Autodesk Inventor part; units mm, degrees
(part 2 of 3)
  line L883 (-85.6699, -58.7455) -> (-80.6699, -50.0853)
  line L884 (-66.3397, -69.9058) -> (-61.3397, -61.2455)
  line L885 (-61.3397, -61.2455) -> (-51.3397, -61.2455)
  line L886 (-51.3397, -61.2455) -> (-46.3397, -69.9058)
  line L887 (-51.3397, -61.2455) -> (-46.3397, -69.9058)
  line L888 (-51.3397, -78.566) -> (-61.3397, -78.566)
  line L889 (-51.3397, -78.566) -> (-61.3397, -78.566)
  line L890 (-61.3397, -78.566) -> (-66.3397, -69.9058)
  line L891 (-61.3397, -78.566) -> (-66.3397, -69.9058)
  line L892 (-46.3397, -69.9058) -> (-51.3397, -78.566)
  line L893 (-47.0096, -58.7455) -> (-42.0096, -50.0853)
  line L894 (-32.0096, -50.0853) -> (-27.0096, -58.7455)
  line L895 (-32.0096, -67.4058) -> (-42.0096, -67.4058)
  line L896 (-27.0096, -58.7455) -> (-32.0096, -67.4058)
  line L897 (-42.0096, -67.4058) -> (-47.0096, -58.7455)
  line L898 (-42.0096, -50.0853) -> (-32.0096, -50.0853)
  line L899 (-12.6795, -78.566) -> (-22.6795, -78.566)
  line L900 (-22.6795, -78.566) -> (-27.6795, -69.9058)
  line L901 (-27.6795, -69.9058) -> (-22.6795, -61.2455)
  line L902 (-7.6795, -69.9058) -> (-12.6795, -78.566)
  line L903 (-12.6795, -61.2455) -> (-7.6795, -69.9058)
  line L904 (-22.6795, -61.2455) -> (-12.6795, -61.2455)
  line L905 (25.981, -56.2455) -> (15.981, -56.2455)
  line L906 (15.981, -61.2455) -> (25.981, -61.2455)
  line L907 (6.6509, -67.4058) -> (-3.3491, -67.4058)
  line L908 (-3.3491, -67.4058) -> (-8.3491, -58.7455)
  line L909 (10.981, -69.9058) -> (15.981, -61.2455)
  line L910 (10.981, -69.9058) -> (15.981, -61.2455)
  line L911 (11.6509, -58.7455) -> (6.6509, -67.4058)
  line L912 (25.981, -61.2455) -> (30.981, -69.9058)
  line L913 (25.981, -61.2455) -> (30.981, -69.9058)
  line L914 (-8.3491, -58.7455) -> (-3.3491, -50.0853)
  line L915 (-3.3491, -50.0853) -> (6.6509, -50.0853)
  line L916 (6.6509, -50.0853) -> (11.6509, -58.7455)
  line L917 (54.6413, -78.566) -> (49.6413, -69.9058)
  line L918 (49.6413, -69.9058) -> (54.6413, -61.2455)
  line L919 (64.6413, -78.566) -> (54.6413, -78.566)
  line L920 (64.6413, -78.566) -> (54.6413, -78.566)
  line L921 (49.6413, -69.9058) -> (54.6413, -61.2455)
  line L922 (35.3111, -67.4058) -> (30.3111, -58.7455)
  line L923 (45.3111, -67.4058) -> (35.3111, -67.4058)
  line L924 (64.6413, -61.2455) -> (69.6413, -69.9058)
  line L925 (50.3111, -58.7455) -> (45.3111, -67.4058)
  line L926 (69.6413, -69.9058) -> (64.6413, -78.566)
  line L927 (73.9714, -72.4058) -> (83.9714, -72.4058)
  line L928 (83.9714, -67.4058) -> (73.9714, -67.4058)
  line L929 (73.9714, -67.4058) -> (68.9714, -58.7455)
  line L930 (45.3111, -50.0853) -> (50.3111, -58.7455)
  line L931 (68.9714, -58.7455) -> (73.9714, -50.0853)
  line L932 (93.3015, -78.566) -> (88.3015, -69.9058)
  line L933 (88.3015, -69.9058) -> (93.3015, -61.2455)
  line L934 (103.3015, -78.566) -> (93.3015, -78.566)
  line L935 (103.3015, -61.2455) -> (108.3015, -69.9058)
  line L936 (108.3015, -69.9058) -> (103.3015, -78.566)
  line L937 (54.6413, -61.2455) -> (64.6413, -61.2455)
  line L938 (73.9714, -50.0853) -> (83.9714, -50.0853)
  line L939 (35.3111, -50.0853) -> (45.3111, -50.0853)
  line L940 (30.3111, -58.7455) -> (35.3111, -50.0853)
  line L941 (15.981, -78.566) -> (10.981, -69.9058)
  line L942 (25.981, -78.566) -> (15.981, -78.566)
  line L943 (25.981, -78.566) -> (15.981, -78.566)
  line L944 (15.981, -78.566) -> (10.981, -69.9058)
  line L945 (69.6413, -69.9058) -> (64.6413, -78.566)
  line L946 (64.6413, -61.2455) -> (69.6413, -69.9058)
  line L947 (35.3111, -72.4058) -> (45.3111, -72.4058)
  line L948 (35.3111, -72.4058) -> (45.3111, -72.4058)
  line L949 (54.6413, -78.566) -> (49.6413, -69.9058)
  line L950 (30.981, -69.9058) -> (25.981, -78.566)
  line L951 (30.981, -69.9058) -> (25.981, -78.566)
  line L952 (103.3015, -56.2455) -> (93.3015, -56.2455)
  line L953 (107.6314, -58.7455) -> (112.6314, -50.0853)
  line L954 (112.6314, -50.0853) -> (122.6314, -50.0853)
  line L955 (112.6314, -67.4058) -> (107.6314, -58.7455)
  line L956 (122.6314, -50.0853) -> (127.6314, -58.7455)
  line L957 (122.6314, -67.4058) -> (112.6314, -67.4058)
  line L958 (127.6314, -58.7455) -> (122.6314, -67.4058)
  line L959 (93.3015, -61.2455) -> (103.3015, -61.2455)
  line L960 (88.9714, -58.7455) -> (83.9714, -67.4058)
  line L961 (83.9714, -50.0853) -> (88.9714, -58.7455)
  line L962 (-109.3301, -72.4063) -> (-104.3301, -81.0665)
  line L963 (-104.3301, -81.0665) -> (-109.3301, -89.7268)
  line L964 (-109.3301, -89.7268) -> (-119.3301, -89.7268)
  line L965 (-119.3301, -72.4063) -> (-109.3301, -72.4063)
  line L966 (-124.3301, -81.0665) -> (-119.3301, -72.4063)
  line L967 (-119.3301, -89.7268) -> (-124.3301, -81.0665)
  line L968 (-105, -92.2268) -> (-100, -83.5665)
  line L969 (-100, -83.5665) -> (-90, -83.5665)
  line L970 (-90, -83.5665) -> (-85, -92.2268)
  line L971 (-85, -92.2268) -> (-90, -100.887)
  line L972 (-90, -100.887) -> (-100, -100.887)
  line L973 (-100, -100.887) -> (-105, -92.2268)
  line L974 (-80.6699, -89.7268) -> (-85.6699, -81.0665)
  line L975 (-65.6699, -81.0665) -> (-70.6699, -89.7268)
  line L976 (-70.6699, -72.4063) -> (-65.6699, -81.0665)
  line L977 (-80.6699, -72.4063) -> (-70.6699, -72.4063)
  line L978 (-70.6699, -89.7268) -> (-80.6699, -89.7268)
  line L979 (-85.6699, -81.0665) -> (-80.6699, -72.4063)
  line L980 (-66.3397, -92.2268) -> (-61.3397, -83.5665)
  line L981 (-61.3397, -83.5665) -> (-51.3397, -83.5665)
  line L982 (-51.3397, -83.5665) -> (-46.3397, -92.2268)
  line L983 (-51.3397, -83.5665) -> (-46.3397, -92.2268)
  line L984 (-51.3397, -100.887) -> (-61.3397, -100.887)
  line L985 (-51.3397, -100.887) -> (-61.3397, -100.887)
  line L986 (-61.3397, -100.887) -> (-66.3397, -92.2268)
  line L987 (-61.3397, -100.887) -> (-66.3397, -92.2268)
  line L988 (-46.3397, -92.2268) -> (-51.3397, -100.887)
  line L989 (-47.0096, -81.0665) -> (-42.0096, -72.4063)
  line L990 (-32.0096, -72.4063) -> (-27.0096, -81.0665)
  line L991 (-32.0096, -89.7268) -> (-42.0096, -89.7268)
  line L992 (-27.0096, -81.0665) -> (-32.0096, -89.7268)
  line L993 (-42.0096, -89.7268) -> (-47.0096, -81.0665)
  line L994 (-42.0096, -72.4063) -> (-32.0096, -72.4063)
  line L995 (-12.6795, -100.887) -> (-22.6795, -100.887)
  line L996 (-22.6795, -100.887) -> (-27.6795, -92.2268)
  line L997 (-27.6795, -92.2268) -> (-22.6795, -83.5665)
  line L998 (-7.6795, -92.2268) -> (-12.6795, -100.887)
  line L999 (-12.6795, -83.5665) -> (-7.6795, -92.2268)
  line L1000 (-22.6795, -83.5665) -> (-12.6795, -83.5665)
  line L1001 (25.981, -78.5665) -> (15.981, -78.5665)
  line L1002 (15.981, -83.5665) -> (25.981, -83.5665)
  line L1003 (6.6509, -89.7268) -> (-3.3491, -89.7268)
  line L1004 (-3.3491, -89.7268) -> (-8.3491, -81.0665)
  line L1005 (10.981, -92.2268) -> (15.981, -83.5665)
  line L1006 (10.981, -92.2268) -> (15.981, -83.5665)
  line L1007 (11.6509, -81.0665) -> (6.6509, -89.7268)
  line L1008 (25.981, -83.5665) -> (30.981, -92.2268)
  line L1009 (25.981, -83.5665) -> (30.981, -92.2268)
  line L1010 (-8.3491, -81.0665) -> (-3.3491, -72.4063)
  line L1011 (-3.3491, -72.4063) -> (6.6509, -72.4063)
  line L1012 (6.6509, -72.4063) -> (11.6509, -81.0665)
  line L1013 (54.6413, -100.887) -> (49.6413, -92.2268)
  line L1014 (49.6413, -92.2268) -> (54.6413, -83.5665)
  line L1015 (64.6413, -100.887) -> (54.6413, -100.887)
  line L1016 (64.6413, -100.887) -> (54.6413, -100.887)
  line L1017 (49.6413, -92.2268) -> (54.6413, -83.5665)
  line L1018 (35.3111, -89.7268) -> (30.3111, -81.0665)
  line L1019 (45.3111, -89.7268) -> (35.3111, -89.7268)
  line L1020 (64.6413, -83.5665) -> (69.6413, -92.2268)
  line L1021 (50.3111, -81.0665) -> (45.3111, -89.7268)
  line L1022 (69.6413, -92.2268) -> (64.6413, -100.887)
  line L1023 (73.9714, -94.7268) -> (83.9714, -94.7268)
  line L1024 (83.9714, -89.7268) -> (73.9714, -89.7268)
  line L1025 (73.9714, -89.7268) -> (68.9714, -81.0665)
  line L1026 (45.3111, -72.4063) -> (50.3111, -81.0665)
  line L1027 (68.9714, -81.0665) -> (73.9714, -72.4063)
  line L1028 (93.3015, -100.887) -> (88.3015, -92.2268)
  line L1029 (88.3015, -92.2268) -> (93.3015, -83.5665)
  line L1030 (103.3015, -100.887) -> (93.3015, -100.887)
  line L1031 (103.3015, -83.5665) -> (108.3015, -92.2268)
  line L1032 (108.3015, -92.2268) -> (103.3015, -100.887)
  line L1033 (54.6413, -83.5665) -> (64.6413, -83.5665)
  line L1034 (73.9714, -72.4063) -> (83.9714, -72.4063)
  line L1035 (35.3111, -72.4063) -> (45.3111, -72.4063)
  line L1036 (30.3111, -81.0665) -> (35.3111, -72.4063)
  line L1037 (15.981, -100.887) -> (10.981, -92.2268)
  line L1038 (25.981, -100.887) -> (15.981, -100.887)
  line L1039 (25.981, -100.887) -> (15.981, -100.887)
  line L1040 (15.981, -100.887) -> (10.981, -92.2268)
  line L1041 (69.6413, -92.2268) -> (64.6413, -100.887)
  line L1042 (64.6413, -83.5665) -> (69.6413, -92.2268)
  line L1043 (35.3111, -94.7268) -> (45.3111, -94.7268)
  line L1044 (35.3111, -94.7268) -> (45.3111, -94.7268)
  line L1045 (54.6413, -100.887) -> (49.6413, -92.2268)
  line L1046 (30.981, -92.2268) -> (25.981, -100.887)
  line L1047 (30.981, -92.2268) -> (25.981, -100.887)
  line L1048 (103.3015, -78.5665) -> (93.3015, -78.5665)
  line L1049 (107.6314, -81.0665) -> (112.6314, -72.4063)
  line L1050 (112.6314, -72.4063) -> (122.6314, -72.4063)
  line L1051 (112.6314, -89.7268) -> (107.6314, -81.0665)
  line L1052 (122.6314, -72.4063) -> (127.6314, -81.0665)
  line L1053 (122.6314, -89.7268) -> (112.6314, -89.7268)
  line L1054 (127.6314, -81.0665) -> (122.6314, -89.7268)
  line L1055 (93.3015, -83.5665) -> (103.3015, -83.5665)
  line L1056 (88.9714, -81.0665) -> (83.9714, -89.7268)
  line L1057 (83.9714, -72.4063) -> (88.9714, -81.0665)
  line L1058 (-109.3301, -94.7273) -> (-104.3301, -103.3875)
  line L1059 (-104.3301, -103.3875) -> (-109.3301, -112.0478)
  line L1060 (-109.3301, -112.0478) -> (-119.3301, -112.0478)
  line L1061 (-119.3301, -94.7273) -> (-109.3301, -94.7273)
  line L1062 (-124.3301, -103.3875) -> (-119.3301, -94.7273)
  line L1063 (-119.3301, -112.0478) -> (-124.3301, -103.3875)
  line L1064 (-105, -114.5478) -> (-100, -105.8875)
  line L1065 (-100, -105.8875) -> (-90, -105.8875)
  line L1066 (-90, -105.8875) -> (-85, -114.5478)
  line L1067 (-85, -114.5478) -> (-90, -123.208)
  line L1068 (-90, -123.208) -> (-100, -123.208)
  line L1069 (-100, -123.208) -> (-105, -114.5478)
  line L1070 (-80.6699, -112.0478) -> (-85.6699, -103.3875)
  line L1071 (-65.6699, -103.3875) -> (-70.6699, -112.0478)
  line L1072 (-70.6699, -94.7273) -> (-65.6699, -103.3875)
  line L1073 (-80.6699, -94.7273) -> (-70.6699, -94.7273)
  line L1074 (-70.6699, -112.0478) -> (-80.6699, -112.0478)
  line L1075 (-85.6699, -103.3875) -> (-80.6699, -94.7273)
  line L1076 (-66.3397, -114.5478) -> (-61.3397, -105.8875)
  line L1077 (-61.3397, -105.8875) -> (-51.3397, -105.8875)
  line L1078 (-51.3397, -105.8875) -> (-46.3397, -114.5478)
  line L1079 (-51.3397, -105.8875) -> (-46.3397, -114.5478)
  line L1080 (-51.3397, -123.208) -> (-61.3397, -123.208)
  line L1081 (-51.3397, -123.208) -> (-61.3397, -123.208)
  line L1082 (-61.3397, -123.208) -> (-66.3397, -114.5478)
  line L1083 (-61.3397, -123.208) -> (-66.3397, -114.5478)
  line L1084 (-46.3397, -114.5478) -> (-51.3397, -123.208)
  line L1085 (-47.0096, -103.3875) -> (-42.0096, -94.7273)
  line L1086 (-32.0096, -94.7273) -> (-27.0096, -103.3875)
  line L1087 (-32.0096, -112.0478) -> (-42.0096, -112.0478)
  line L1088 (-27.0096, -103.3875) -> (-32.0096, -112.0478)
  line L1089 (-42.0096, -112.0478) -> (-47.0096, -103.3875)
  line L1090 (-42.0096, -94.7273) -> (-32.0096, -94.7273)
  line L1091 (-12.6795, -123.208) -> (-22.6795, -123.208)
  line L1092 (-22.6795, -123.208) -> (-27.6795, -114.5478)
  line L1093 (-27.6795, -114.5478) -> (-22.6795, -105.8875)
  line L1094 (-7.6795, -114.5478) -> (-12.6795, -123.208)
  line L1095 (-12.6795, -105.8875) -> (-7.6795, -114.5478)
  line L1096 (-22.6795, -105.8875) -> (-12.6795, -105.8875)
  line L1097 (25.981, -100.8875) -> (15.981, -100.8875)
  line L1098 (15.981, -105.8875) -> (25.981, -105.8875)
  line L1099 (6.6509, -112.0478) -> (-3.3491, -112.0478)
  line L1100 (-3.3491, -112.0478) -> (-8.3491, -103.3875)
  line L1101 (10.981, -114.5478) -> (15.981, -105.8875)
  line L1102 (10.981, -114.5478) -> (15.981, -105.8875)
  line L1103 (11.6509, -103.3875) -> (6.6509, -112.0478)
  line L1104 (25.981, -105.8875) -> (30.981, -114.5478)
  line L1105 (25.981, -105.8875) -> (30.981, -114.5478)
  line L1106 (-8.3491, -103.3875) -> (-3.3491, -94.7273)
  line L1107 (-3.3491, -94.7273) -> (6.6509, -94.7273)
  line L1108 (6.6509, -94.7273) -> (11.6509, -103.3875)
  line L1109 (54.6413, -123.208) -> (49.6413, -114.5478)
  line L1110 (49.6413, -114.5478) -> (54.6413, -105.8875)
  line L1111 (64.6413, -123.208) -> (54.6413, -123.208)
  line L1112 (64.6413, -123.208) -> (54.6413, -123.208)
  line L1113 (49.6413, -114.5478) -> (54.6413, -105.8875)
  line L1114 (35.3111, -112.0478) -> (30.3111, -103.3875)
  line L1115 (45.3111, -112.0478) -> (35.3111, -112.0478)
  line L1116 (64.6413, -105.8875) -> (69.6413, -114.5478)
  line L1117 (50.3111, -103.3875) -> (45.3111, -112.0478)
  line L1118 (69.6413, -114.5478) -> (64.6413, -123.208)
  line L1119 (73.9714, -117.0478) -> (83.9714, -117.0478)
  line L1120 (83.9714, -112.0478) -> (73.9714, -112.0478)
  line L1121 (73.9714, -112.0478) -> (68.9714, -103.3875)
  line L1122 (45.3111, -94.7273) -> (50.3111, -103.3875)
  line L1123 (68.9714, -103.3875) -> (73.9714, -94.7273)
  line L1124 (93.3015, -123.208) -> (88.3015, -114.5478)
  line L1125 (88.3015, -114.5478) -> (93.3015, -105.8875)
  line L1126 (103.3015, -123.208) -> (93.3015, -123.208)
  line L1127 (103.3015, -105.8875) -> (108.3015, -114.5478)
  line L1128 (108.3015, -114.5478) -> (103.3015, -123.208)
  line L1129 (54.6413, -105.8875) -> (64.6413, -105.8875)
  line L1130 (73.9714, -94.7273) -> (83.9714, -94.7273)
  line L1131 (35.3111, -94.7273) -> (45.3111, -94.7273)
  line L1132 (30.3111, -103.3875) -> (35.3111, -94.7273)
  line L1133 (15.981, -123.208) -> (10.981, -114.5478)
  line L1134 (25.981, -123.208) -> (15.981, -123.208)
  line L1135 (25.981, -123.208) -> (15.981, -123.208)
  line L1136 (15.981, -123.208) -> (10.981, -114.5478)
  line L1137 (69.6413, -114.5478) -> (64.6413, -123.208)
  line L1138 (64.6413, -105.8875) -> (69.6413, -114.5478)
  line L1139 (35.3111, -117.0478) -> (45.3111, -117.0478)
  line L1140 (35.3111, -117.0478) -> (45.3111, -117.0478)
  line L1141 (54.6413, -123.208) -> (49.6413, -114.5478)
  line L1142 (30.981, -114.5478) -> (25.981, -123.208)
  line L1143 (30.981, -114.5478) -> (25.981, -123.208)
  line L1144 (103.3015, -100.8875) -> (93.3015, -100.8875)
  line L1145 (107.6314, -103.3875) -> (112.6314, -94.7273)
  line L1146 (112.6314, -94.7273) -> (122.6314, -94.7273)
  line L1147 (112.6314, -112.0478) -> (107.6314, -103.3875)
  line L1148 (122.6314, -94.7273) -> (127.6314, -103.3875)
  line L1149 (122.6314, -112.0478) -> (112.6314, -112.0478)
  line L1150 (127.6314, -103.3875) -> (122.6314, -112.0478)
  line L1151 (93.3015, -105.8875) -> (103.3015, -105.8875)
  line L1152 (88.9714, -103.3875) -> (83.9714, -112.0478)
  line L1153 (83.9714, -94.7273) -> (88.9714, -103.3875)
  point P0 (0, 0)
  point P1 (-100, 79)
  point P2 (-100, 71.25)
  point P3 (-100, 86.75)
  point P4 (-60, 79)
  point P5 (-60, 71.25)
  point P6 (-60, 86.75)
  point P7 (-20, 79)
  point P8 (-20, 71.25)
  point P9 (-20, 86.75)
  point P10 (20, 79)
  point P11 (20, 71.25)
  point P12 (20, 86.75)
  point P13 (60, 79)
  point P14 (60, 71.25)
  point P15 (60, 86.75)
  point P16 (100, 79)
  point P17 (100, 71.25)
  point P18 (100, 86.75)
  point P19 (100, 79)
  point P20 (-80, 39.5)
  point P21 (-80, 47.25)
  point P22 (-80, 31.75)
  point P23 (-40, 47.25)
  point P24 (-40, 39.5)
  point P25 (-40, 31.75)
  point P26 (0, 47.25)
  point P27 (0, 39.5)
  point P28 (0, 31.75)
  point P29 (40, 47.25)
  point P30 (40, 39.5)
  point P31 (40, 31.75)
  point P32 (80, 47.25)
  point P33 (80, 39.5)
  point P34 (80, 31.75)
  point P35 (-100, 0)
  point P36 (-100, -7.75)
  point P37 (-100, 7.75)
  point P38 (-60, 0)
  point P39 (-60, -7.75)
  point P40 (-60, 7.75)
  point P41 (-20, 0)
  point P42 (-20, -7.75)
  point P43 (-20, 7.75)
  point P44 (20, 0)
  point P45 (20, -7.75)
  point P46 (20, 7.75)
  point P47 (60, 0)
  point P48 (60, -7.75)
  point P49 (60, 7.75)
  point P50 (100, 0)
  point P51 (100, 0)
  point P52 (100, -7.75)
  point P53 (100, 7.75)
  point P54 (-100, -79)
  point P55 (-100, -86.75)
  point P56 (-100, -71.25)
  point P57 (-60, -79)
  point P58 (-60, -86.75)
  point P59 (-60, -71.25)
  point P60 (-20, -79)
  point P61 (-20, -86.75)
  point P62 (-20, -71.25)
  point P63 (20, -79)
  point P64 (20, -86.75)
  point P65 (20, -71.25)
  point P66 (60, -79)
  point P67 (60, -86.75)
  point P68 (60, -71.25)
  point P69 (100, -79)
  point P70 (100, -79)
  point P71 (100, -86.75)
  point P72 (100, -71.25)
  point P73 (-80, -39.5)
  point P74 (-80, -47.25)
  point P75 (-80, -31.75)
  point P76 (0, -31.75)
  point P77 (0, -39.5)
  point P78 (0, -47.25)
  point P79 (40, -31.75)
  point P80 (40, -39.5)
  point P81 (40, -47.25)
  point P82 (80, -31.75)
  point P83 (80, -39.5)
  point P84 (80, -47.25)
  point P85 (-40, -31.75)
  point P86 (-40, -39.5)
  point P87 (-40, -47.25)
  point P88 (100, -86.75)
  point P89 (-60, -86.75)
  point P90 (60, 79)
  point P91 (-95, 86.3397)
  point P92 (-95, 95)
  point P93 (-75.6699, 75.1795)
  point P94 (-75.6699, 83.8397)
  point P95 (-75.6699, 97.5)
  point P96 (-174.6517, 120.5465)
  point P97 (-114.3301, 97.5)
  point P98 (-95, 108.6603)
  point P99 (-102.5, 68.3494)
  point P100 (-83.1699, 48.5289)
  point P101 (-56.3397, 55.359)
  point P102 (-48.8397, 82.0096)
  point P103 (-68.1699, 101.8301)
  point P104 (-114.3301, 75.1795)
  point P105 (-37.0096, 75.1795)
  point P106 (-44.5096, 70.8494)
  point P107 (-29.5096, 48.5289)
  point P108 (-10.1795, 68.3494)
  point P109 (-17.6795, 95)
  point P110 (-44.5096, 101.8301)
  point P111 (20.981, 95)
  point P112 (40.3111, 75.1795)
  point P113 (32.8111, 48.5289)
  point P114 (40.3111, 83.8397)
  point P115 (40.3111, 97.5)
  point P116 (47.8111, 101.8301)
  point P117 (13.481, 68.3494)
  point P118 (20.981, 108.6603)
  point P119 (1.6509, 75.1795)
  point P120 (1.6509, 97.5)
  point P121 (59.6413, 55.359)
  point P122 (67.1413, 82.0096)
  point P123 (71.4714, 101.8301)
  point P124 (78.9714, 75.1795)
  point P125 (71.4714, 70.8494)
  point P126 (86.4714, 48.5289)
  point P127 (98.3015, 95)
  point P128 (105.8015, 68.3494)
  point P129 (117.6314, 75.1795)
  point P130 (98.3014, 33.0387)
  point P131 (98.3014, 41.6989)
  point P132 (144.4614, 37.3688)
  point P133 (136.9614, 41.6989)
  point P134 (163.7914, 79.5096)
  point P135 (156.2914, 75.1795)
  point P136 (136.9614, 117.3203)
  point P137 (136.9614, 108.66)
  point P138 (90.8014, 112.9902)
  point P139 (98.3014, 108.66)
  point P140 (70, 33.038)
  point P141 (86.4714, -18.4331)
  point P142 (93.3014, -16.6028)
  point P143 (103.3014, -16.6028)
  point P144 (78.9714, 8.2175)
  point P145 (71.4714, 3.8874)
  point P146 (59.6413, -11.603)
  point P147 (105.8015, 1.3874)
  point P148 (100, 12.038)
  point P149 (117.6314, 8.2175)
  point P150 (67.1413, 15.0476)
  point P151 (32.8111, -18.4331)
  point P152 (40.3111, 8.2175)
  point P153 (13.481, 1.3874)
  point P154 (98.3014, 41.698)
  point P155 (98.3015, 28.038)
  point P156 (40.3111, 16.8777)
  point P157 (71.4714, 34.8681)
  point P158 (90.8014, 46.0282)
  point P159 (40.3111, 30.538)
  point P160 (47.8111, 34.8681)
  point P161 (20.981, 28.038)
  point P162 (20.981, 41.6983)
  point P163 (-48.8397, 15.0476)
  point P164 (1.6509, 8.2175)
  point P165 (-83.1699, -18.4331)
  point P166 (-29.5096, -18.4331)
  point P167 (1.6509, 30.538)
  point P168 (-10.1795, 1.3874)
  point P169 (-44.5096, 3.8874)
  point P170 (-37.0096, 8.2175)
  point P171 (-17.6795, 28.038)
  point P172 (-44.5096, 34.8681)
  point P173 (-68.1699, 34.8681)
  point P174 (-75.6699, 8.2175)
  point P175 (-56.3397, -11.603)
  point P176 (-75.6699, 30.538)
  point P177 (-75.6699, 16.8777)
  point P178 (-95, 28.038)
  point P179 (-95, 19.3777)
  point P180 (-95, 41.6983)
  point P181 (-102.5, 1.3874)
  point P182 (-114.3301, 8.2175)
  point P183 (-114.3301, 30.538)
  point P184 (0, -66.962)
  point P185 (-56.3399, 41.6985)
  point P186 (-17.6795, 41.6985)
  point P187 (1.6509, 52.859)
  point P188 (59.6413, 41.6983)
  point P189 (-68.1699, 48.5289)
  point P190 (-114.3301, 52.859)
  point P191 (-114.3301, -14.1035)
  point P192 (-102.5, -20.9336)
  point P193 (-75.6699, -14.1035)
  point P194 (-75.6699, -5.4433)
  point P195 (-56.3397, -33.924)
  point P196 (-44.5096, -18.4336)
  point P197 (-37.0096, -14.1035)
  point P198 (-46.3397, -2.9433)
  point P199 (-46.3397, -2.9433)
  dimension "d0" = 220
  dimension "d1" = 200
  dimension "d2" = 5.5
  dimension "d3" = 15.5
  dimension "d7" = 10
  dimension "d8" = 21
  dimension "d13" = 40
  dimension "d20" = 5.5
  dimension "d21" = 15.5
  dimension "d22" = 30
  dimension "d24" = 55
  dimension "d30" = 40
  dimension "d37" = 79
  dimension "d44" = 79
  dimension "d51" = 13.25
  dimension "d52" = 13.25
  dimension "d76" = 180
  dimension "d77" = 10
  dimension "d159" = 20
  dimension "d160" = 5
  dimension "d161" = 5
  dimension "d162" = 20
  dimension "d164" = 5
  dimension "d166" = 20
  dimension "d167" = 5
  dimension "d168" = 5
  dimension "d170" = 20
  dimension "d171" = 5
  dimension "d172" = 20
  dimension "d173" = 5
  dimension "d174" = 5
  dimension "d175" = 5
  dimension "d178" = 360
  dimension "d182" = 60
  dimension "d184" = 20
  dimension "d185" = 5
  dimension "d186" = 5
  dimension "d189" = 240
  dimension "d193" = 115.981
  dimension "d198" = 20
  dimension "d199" = 38.6602
  dimension "d200" = 38.66
  dimension "d203" = 360
  dimension "d207" = 66.962
  dimension "d212" = 5.0005
  dimension "d213" = 20
  dimension "d214" = 5
  dimension "d215" = 5
  dimension "d216" = 20
  dimension "d217" = 20
  dimension "d218" = 20
  dimension "d219" = 20
  dimension "d222" = 22.321
  constraints: 2358 end point, 1202 vertical alignment, 738 parallel, 118 point on circle, 56 centre point, 51 collinear, 34 equal radius, 18 horizontal, 10 midpoint, 8 tangent, 6 horizontal alignment, 4 vertical, 1 perpendicular, 1 point on line, 899 other
  measures "d0" distance of L1.end L2.end
  measures "d1" distance of L1.start L1.end
  measures "d2" distance between parallel lines of L8 L7
  measures "d3" distance of point (-100, 71.25) point (-100, 86.75)
  measures "d8" distance from line of L2 point (-100, 79)
  measures "d13" distance of L7.start L9.start
  measures "d20" distance between parallel lines of L26 L25
  measures "d21" distance of point (-80, 47.25) point (-80, 31.75)
  measures "d24" vertical distance of point (-80, 31.75) point (-100, 86.75)
  measures "d30" distance of point (-80, 47.25) point (-40, 47.25)
  measures "d37" distance of point (-100, 79) point (-100, 0)
  measures "d44" distance of L24.start L75.start
  measures "d52" distance from line of L2 point (-100, 86.75)
  measures "d77" distance from line of L90 point (60, 79)
  measures "d159" distance of L91.start L93.end
  measures "d161" distance from line of L2 point (-95, 95)
  measures "d162" distance of L100.end L97.end
  measures "d164" distance between parallel lines of L91 L98
  measures "d166" distance of L105.start L107.end
  measures "d167" distance between parallel lines of L107 L96
  measures "d168" distance between parallel lines of L99 L106
  measures "d170" distance of L121.end L117.end
  measures "d171" distance between parallel lines of L94 L119
  measures "d172" distance of L125.start L123.end
  measures "d173" distance between parallel lines of L95 L124
  measures "d174" distance between parallel lines of L108 L125
  measures "d175" distance between parallel lines of L123 L121
  measures "d184" distance of L197.start L195.end
  measures "d185" distance from line of point (-44.51, 70.849) L154
  measures "d186" distance between parallel lines of L200 L187
  measures "d193" distance of L107.end L245.end
  measures "d198" distance of L353.start L351.end
  measures "d199" distance of point (40.311, 75.179) point (78.971, 75.179)
  measures "d200" distance of point (117.631, 75.179) point (78.971, 75.179)
  measures "d207" distance of L1.end L626.end
  measures "d212" distance between parallel lines of L130 L603
  measures "d213" distance of L646.start L644.end
  measures "d214" distance from line of point (-68.17, 48.529) L649
  measures "d215" distance between parallel lines of L565 L644
  measures "d216" distance of L652.start L650.end
  measures "d217" distance of L658.start L656.end
  measures "d218" distance of L662.end L664.start
  measures "d219" distance of L670.start L668.end
  measures "d222" distance of L609.start L674.start
extrude "돌출1" add sketch "스케치1" along normal blind 5 contours L3 L1061 L1058 L0 | L1058 L1061 L3 L964 L963 L962 L965 L868 L867 L866 L869 L772 L771 L770 L773 L676 L675 L674 L677 L608 L607 L609 L610 L615 L614 L613 L387 L583 L584 L588 L564 L565 L562 L560 L557 L558 L559 L537 L539 L538 L536 L535 L486 L465 L464 L484 L488 L90 L472 L473 L435 L396 L391 L390 L835 L833 L931 L929 L1027 L1025 L0 L1022 L1020 L1033 L71 L919 L926 L924 L937 L918 L917 L69 L1014 L1013 L1122 L1043 L1132 L1046 L1008 L1002 L68 L942 L950 L912 L906 L909 L941 L66 L1005 L1037 L1108 L1107 L1106 L998 L999 L1000 L65 L899 L902 L903 L904 L901 L900 L63 L997 L996 L1086 L1090 L1085 L988 L982 L981 L62 L888 L892 L886 L885 L884 L890 L60 A37 L980 L986 L1072 L1073 L1075 L971 L970 L969 L59 L876 L875 L874 L873 L872 L877 A35 L58 A34 L968 L973 | L3 L965 L962 L963 L964 | L1075 L1073 L1072 L0 | A34 L58 A35 L877 L876 L59 L969 L968 | L3 L869 L866 L867 L868 | L3 L773 L770 L771 L772 | L1085 L1090 L1086 L0 | A37 L60 L890 L888 L62 L981 L980 | L3 L677 L674 L675 L676 | L3 L610 L609 L607 L608 | L1106 L1107 L1108 L0 | L63 L900 L899 L65 L1000 L997 | L3 L387 L613 L614 L615 | L3 L616 L613 L387 | L3 L669 L670 L672 L671 L191 L190 L189 L194 L118 L119 L121 L2 L108 L107 L106 L105 L110 L222 L223 L224 L219 L220 L290 L289 L291 L293 L294 L246 L245 L244 L243 L248 L90 L323 L321 L322 L330 L331 L332 L387 L664 L666 L665 L667 L662 L488 L487 L35 L240 L236 L257 L260 L255 L238 L33 L486 L502 L501 L500 L496 L495 L535 L540 L32 L657 L658 L660 L659 L661 L656 L30 L537 L652 L654 L653 L655 L650 L559 L561 L29 L203 L204 L205 L206 L201 L202 A14 L27 L562 L646 L648 L647 L649 L644 L565 L590 L25 L143 L142 L141 L146 L145 L144 A13 L26 L583 L600 L602 L603 L604 L601 L613 L616 | L3 L671 L672 L670 L669 | L1132 L1043 L1122 L0 | L66 L942 L68 L1002 | L3 L194 L189 L190 L191 | L26 A13 L144 L143 L25 L590 L583 | L3 L2 L121 L119 L118 | L90 L1025 L1024 L1056 L1057 L927 L1027 L929 L928 L960 L961 L831 L931 L833 L832 A53 L864 L865 L735 L835 L390 L389 L388 L418 L392 L391 L396 L394 L417 L416 L476 L435 L473 L475 L477 L479 L387 L359 L1 L427 L428 L761 L763 L857 L859 L953 L955 L1049 L1051 L1145 L0 L1032 L1031 L1055 L74 L934 L936 L935 L959 L933 L932 L72 L1029 L1028 L1153 L1023 L1123 | L1123 L1023 L1153 L0 | L69 L919 L71 L1033 | L27 A14 L202 L203 L29 L561 L562 | L72 L934 L74 L1055 | L832 A53 | L30 L657 L32 L540 | L90 L332 L337 L36 L474 L472 L387 | L90 L330 L334 L333 L324 L325 L322 L321 L326 L327 L329 L2 L1 L356 L351 L387 L360 L361 L362 L357 L358 L479 L474 L38 L337 L338 L336 L335 L331 | L36 L337 L38 L474 | L33 L240 L35 L487 | L7 L93 L92 L8 A0 L133 L132 | L9 L170 L169 L11 A2 L153 L158 | L12 L218 L213 L14 A4 L211 | L15 L295 L17 A6 L296 | L18 L313 L20 A8 L302 | L21 L341 L23 A10 L349 | L40 A23 L641 L642 | L42 A24 L637 L638 | A27 L634 | A29 L630 | A31 L628 | A33 L625 | A46 L77 L782 L786 | A49 L811 | A51 L827 | L801 L799 A55 L87
sketch "스케치2" plane through (0, 0, 0) normal (0, 0, -1) x (-1, 0, 0)
  line L0 (-70, 99.2816) -> (-70, 100) projected
  line L1 (-103.8136, -100) -> (-54.1291, -100) projected
  line L2 (-70, 100) -> (110, 100)
  line L3 (110, 100) -> (110, -100)
  line L4 (110, -100) -> (-70, -100)
  line L5 (-70, -100) -> (-70, 100)
  line L6 (105, 95) -> (-65, 95)
  line L7 (-65, 95) -> (-65, -95)
  line L8 (-65, -95) -> (105, -95)
  line L9 (105, -95) -> (105, 95)
  line L10 (-12.5, 95) -> (-12.5, -95)
  line L11 (-17.25, -78.5665) -> (-17.25, -78.566) projected
  line L12 (-7.5, -95) -> (-7.5, 95)
  line L13 (-2.75, -34.5) -> (-2.75, -44.5) projected
  line L14 (47.5, -95) -> (47.5, 95)
  line L15 (52.5, -95) -> (52.5, 95)
  line L16 (57.25, -74) -> (57.25, -84) projected
  line L17 (42.75, -44.5) -> (42.75, -43.8024) projected
  line L18 (12.6795, -78.566) -> (22.6795, -78.566) projected
  line L19 (7.6795, -69.9058) -> (12.6795, -78.566) projected
  line L20 (12.6795, -61.2455) -> (7.6795, -69.9058) projected
  line L21 (22.6795, -61.2455) -> (12.6795, -61.2455) projected
  line L22 (27.6795, -69.9058) -> (22.6795, -61.2455) projected
  line L23 (22.6795, -78.566) -> (27.6795, -69.9058) projected
  line L24 (51.3397, -78.566) -> (61.3397, -78.566) projected
  line L25 (46.3397, -69.9058) -> (51.3397, -78.566) projected
  line L26 (51.3397, -61.2455) -> (46.3397, -69.9058) projected
  line L27 (61.3397, -61.2455) -> (51.3397, -61.2455) projected
  line L28 (66.3397, -69.9058) -> (61.3397, -61.2455) projected
  line L29 (61.3397, -78.566) -> (66.3397, -69.9058) projected
  line L30 (-73.9714, -0.4428) -> (-68.9714, 8.2175) projected
  line L31 (-83.9714, -0.4428) -> (-73.9714, -0.4428) projected
  line L32 (-88.9714, 8.2175) -> (-83.9714, -0.4428) projected
  line L33 (-83.9714, 16.8777) -> (-88.9714, 8.2175) projected
  line L34 (-73.9714, 16.8777) -> (-83.9714, 16.8777) projected
  line L35 (-68.9714, 8.2175) -> (-73.9714, 16.8777) projected
  line L36 (-83.9714, 44.1987) -> (-73.9714, 44.1987) projected
  line L37 (-88.9714, 52.859) -> (-83.9714, 44.1987) projected
  line L38 (-83.9714, 61.5192) -> (-88.9714, 52.859) projected
  line L39 (-73.9714, 61.5192) -> (-83.9714, 61.5192) projected
  line L40 (-68.9714, 52.859) -> (-73.9714, 61.5192) projected
  line L41 (-73.9714, 44.1987) -> (-68.9714, 52.859) projected
  line L42 (-73.9714, -89.7268) -> (-68.9714, -81.0665) projected
  line L43 (-83.9714, -89.7268) -> (-73.9714, -89.7268) projected
  line L44 (-88.9714, -81.0665) -> (-83.9714, -89.7268) projected
  line L45 (-83.9714, -72.4063) -> (-88.9714, -81.0665) projected
  line L46 (-73.9714, -72.4063) -> (-83.9714, -72.4063) projected
  line L47 (-68.9714, -81.0665) -> (-73.9714, -72.4063) projected
  line L48 (-73.9714, -67.4058) -> (-68.9714, -58.7455) projected
  line L49 (-83.9714, -67.4058) -> (-73.9714, -67.4058) projected
  line L50 (-88.9714, -58.7455) -> (-83.9714, -67.4058) projected
  line L51 (-83.9714, -50.0853) -> (-88.9714, -58.7455) projected
  line L52 (-73.9714, -50.0853) -> (-83.9714, -50.0853) projected
  line L53 (-68.9714, -58.7455) -> (-73.9714, -50.0853) projected
  line L54 (-73.9714, -45.0848) -> (-68.9714, -36.4245) projected
  line L55 (-83.9714, -45.0848) -> (-73.9714, -45.0848) projected
  line L56 (-88.9714, -36.4245) -> (-83.9714, -45.0848) projected
  line L57 (-83.9714, -27.7643) -> (-88.9714, -36.4245) projected
  line L58 (-73.9714, -27.7643) -> (-83.9714, -27.7643) projected
  line L59 (-68.9714, -36.4245) -> (-73.9714, -27.7643) projected
  line L60 (-68.9714, -14.103) -> (-73.9714, -5.4428) projected
  line L61 (-68.9715, -14.1033) -> (-68.9714, -14.103) projected
  line L62 (-68.9714, -14.1035) -> (-68.9715, -14.1033) projected
  line L63 (-73.9714, -22.7638) -> (-68.9714, -14.1035) projected
  line L64 (-83.9714, -22.7638) -> (-73.9714, -22.7638) projected
  line L65 (-88.9714, -14.1035) -> (-83.9714, -22.7638) projected
  line L66 (-88.9712, -14.1033) -> (-88.9714, -14.1035) projected
  line L67 (-88.9714, -14.103) -> (-88.9712, -14.1033) projected
  line L68 (-83.9714, -5.4428) -> (-88.9714, -14.103) projected
  line L69 (-73.9714, -5.4428) -> (-83.9714, -5.4428) projected
  line L70 (90, -78.566) -> (100, -78.566) projected
  line L71 (85, -69.9058) -> (90, -78.566) projected
  line L72 (90, -61.2455) -> (85, -69.9058) projected
  line L73 (100, -61.2455) -> (90, -61.2455) projected
  line L74 (105, -69.9058) -> (100, -61.2455) projected
  line L75 (100, -78.566) -> (105, -69.9058) projected
  line L76 (-64.6413, 33.038) -> (-54.6413, 33.038) projected
  line L77 (-69.6413, 41.6983) -> (-64.6413, 33.038) projected
  line L78 (-64.6413, 50.3585) -> (-69.6413, 41.6983) projected
  line L79 (-54.6413, 50.3585) -> (-64.6413, 50.3585) projected
  line L80 (-49.6413, 41.6983) -> (-54.6413, 50.3585) projected
  line L81 (-54.6413, 33.038) -> (-49.6413, 41.6983) projected
  line L82 (-45.3111, 44.1987) -> (-35.3111, 44.1987) projected
  line L83 (-50.3111, 52.859) -> (-45.3111, 44.1987) projected
  line L84 (-45.3111, 61.5192) -> (-50.3111, 52.859) projected
  line L85 (-35.3111, 61.5192) -> (-45.3111, 61.5192) projected
  line L86 (-30.3111, 52.859) -> (-35.3111, 61.5192) projected
  line L87 (-35.3111, 44.1987) -> (-30.3111, 52.859) projected
  line L88 (-25.981, 33.038) -> (-15.981, 33.038) projected
  line L89 (-30.981, 41.6983) -> (-25.981, 33.038) projected
  line L90 (-25.981, 50.3585) -> (-30.981, 41.6983) projected
  line L91 (-15.981, 50.3585) -> (-25.981, 50.3585) projected
  line L92 (-10.981, 41.6983) -> (-15.981, 50.3585) projected
  line L93 (-15.981, 33.038) -> (-10.981, 41.6983) projected
  line L94 (3.3491, 39.1983) -> (-6.6509, 39.1983) projected
  line L95 (8.3491, 30.538) -> (3.3491, 39.1983) projected
  line L96 (3.3491, 21.8777) -> (8.3491, 30.538) projected
  line L97 (-6.6509, 21.8777) -> (3.3491, 21.8777) projected
  line L98 (-11.6509, 30.538) -> (-6.6509, 21.8777) projected
  line L99 (-6.6509, 39.1983) -> (-11.6509, 30.538) projected
  line L100 (32.0096, 44.1987) -> (42.0096, 44.1987) projected
  line L101 (27.0096, 52.859) -> (32.0096, 44.1987) projected
  line L102 (32.0096, 61.5192) -> (27.0096, 52.859) projected
  line L103 (42.0096, 61.5192) -> (32.0096, 61.5192) projected
  line L104 (47.0096, 52.859) -> (42.0096, 61.5192) projected
  line L105 (42.0096, 44.1987) -> (47.0096, 52.859) projected
  line L106 (70.6699, 44.1987) -> (80.6699, 44.1987) projected
  line L107 (65.6699, 52.859) -> (70.6699, 44.1987) projected
  line L108 (70.6699, 61.5192) -> (65.6699, 52.859) projected
  line L109 (80.6699, 61.5192) -> (70.6699, 61.5192) projected
  line L110 (85.6699, 52.859) -> (80.6699, 61.5192) projected
  line L111 (80.6699, 44.1987) -> (85.6699, 52.859) projected
  line L112 (32.0096, -5.4428) -> (27.0096, -14.103) projected
  line L113 (42.0096, -5.4428) -> (32.0096, -5.4428) projected
  line L114 (47.0096, -14.103) -> (42.0096, -5.4428) projected
  line L115 (47.0095, -14.1033) -> (47.0096, -14.103) projected
  line L116 (47.0096, -14.1035) -> (47.0095, -14.1033) projected
  line L117 (42.0096, -22.7638) -> (47.0096, -14.1035) projected
  line L118 (32.0096, -22.7638) -> (42.0096, -22.7638) projected
  line L119 (27.0096, -14.1035) -> (32.0096, -22.7638) projected
  line L120 (27.0098, -14.1033) -> (27.0096, -14.1035) projected
  line L121 (27.0096, -14.103) -> (27.0098, -14.1033) projected
  line L122 (27.6795, -2.9428) -> (22.6795, 5.7175) projected
  line L123 (22.6795, -11.603) -> (27.6795, -2.9428) projected
  line L124 (12.6795, -11.603) -> (22.6795, -11.603) projected
  line L125 (7.6795, -2.9428) -> (12.6795, -11.603) projected
  line L126 (12.6795, 5.7175) -> (7.6795, -2.9428) projected
  line L127 (22.6795, 5.7175) -> (12.6795, 5.7175) projected
  line L128 (-64.6413, 10.7175) -> (-54.6413, 10.7175) projected
  line L129 (-69.6413, 19.3777) -> (-64.6413, 10.7175) projected
  line L130 (-64.6413, 28.038) -> (-69.6413, 19.3777) projected
  line L131 (-54.6413, 28.038) -> (-64.6413, 28.038) projected
  line L132 (-49.6413, 19.3777) -> (-54.6413, 28.038) projected
  line L133 (-54.6413, 10.7175) -> (-49.6413, 19.3777) projected
  line L134 (-25.981, 10.7175) -> (-15.981, 10.7175) projected
  line L135 (-30.981, 19.3777) -> (-25.981, 10.7175) projected
  line L136 (-25.981, 28.038) -> (-30.981, 19.3777) projected
  line L137 (-15.981, 28.038) -> (-25.981, 28.038) projected
  line L138 (-10.981, 19.3777) -> (-15.981, 28.038) projected
  line L139 (-15.981, 10.7175) -> (-10.981, 19.3777) projected
  line L140 (61.3397, 10.7175) -> (66.3397, 19.3777) projected
  line L141 (51.3397, 10.7175) -> (61.3397, 10.7175) projected
  line L142 (46.3397, 19.3777) -> (51.3397, 10.7175) projected
  line L143 (51.3397, 28.038) -> (46.3397, 19.3777) projected
  line L144 (61.3397, 28.038) -> (51.3397, 28.038) projected
  line L145 (66.3397, 19.3777) -> (61.3397, 28.038) projected
  line L146 (100, 10.7175) -> (105, 19.3777) projected
  line L147 (90, 10.7175) -> (100, 10.7175) projected
  line L148 (85, 19.3777) -> (90, 10.7175) projected
  line L149 (90, 28.038) -> (85, 19.3777) projected
  line L150 (100, 28.038) -> (90, 28.038) projected
  line L151 (105, 19.3777) -> (100, 28.038) projected
  line L152 (80.6699, -22.7638) -> (85.6699, -14.1035) projected
  line L153 (70.6699, -22.7638) -> (80.6699, -22.7638) projected
  line L154 (65.6699, -14.1035) -> (70.6699, -22.7638) projected
  line L155 (65.67, -14.1033) -> (65.6699, -14.1035) projected
  line L156 (65.6699, -14.103) -> (65.67, -14.1033) projected
  line L157 (70.6699, -5.4428) -> (65.6699, -14.103) projected
  line L158 (80.6699, -5.4428) -> (70.6699, -5.4428) projected
  line L159 (85.6699, -14.103) -> (80.6699, -5.4428) projected
  line L160 (85.6697, -14.1033) -> (85.6699, -14.103) projected
  line L161 (85.6699, -14.1035) -> (85.6697, -14.1033) projected
  line L162 (61.3397, -16.6035) -> (51.3397, -16.6035) projected
  line L163 (66.3397, -25.2638) -> (61.3397, -16.6035) projected
  line L164 (61.3397, -33.924) -> (66.3397, -25.2638) projected
  line L165 (51.3397, -33.924) -> (61.3397, -33.924) projected
  line L166 (46.3397, -25.2638) -> (51.3397, -33.924) projected
  line L167 (51.3397, -16.6035) -> (46.3397, -25.2638) projected
  line L168 (-15.981, -16.6035) -> (-25.981, -16.6035) projected
  line L169 (-10.981, -25.2638) -> (-15.981, -16.6035) projected
  line L170 (-15.981, -33.924) -> (-10.981, -25.2638) projected
  line L171 (-25.981, -33.924) -> (-15.981, -33.924) projected
  line L172 (-30.981, -25.2638) -> (-25.981, -33.924) projected
  line L173 (-25.981, -16.6035) -> (-30.981, -25.2638) projected
  line L174 (-35.3111, -22.7638) -> (-30.3111, -14.1035) projected
  line L175 (-45.3111, -22.7638) -> (-35.3111, -22.7638) projected
  line L176 (-50.3111, -14.1035) -> (-45.3111, -22.7638) projected
  line L177 (-50.311, -14.1033) -> (-50.3111, -14.1035) projected
  line L178 (-50.3111, -14.103) -> (-50.311, -14.1033) projected
  line L179 (-45.3111, -5.4428) -> (-50.3111, -14.103) projected
  line L180 (-35.3111, -5.4428) -> (-45.3111, -5.4428) projected
  line L181 (-30.3111, -14.103) -> (-35.3111, -5.4428) projected
  line L182 (-30.3113, -14.1033) -> (-30.3111, -14.103) projected
  line L183 (-30.3111, -14.1035) -> (-30.3113, -14.1033) projected
  line L184 (-54.6413, -16.6035) -> (-64.6413, -16.6035) projected
  line L185 (-49.6413, -25.2638) -> (-54.6413, -16.6035) projected
  line L186 (-54.6413, -33.924) -> (-49.6413, -25.2638) projected
  line L187 (-64.6413, -33.924) -> (-54.6413, -33.924) projected
  line L188 (-69.6413, -25.2638) -> (-64.6413, -33.924) projected
  line L189 (-64.6413, -16.6035) -> (-69.6413, -25.2638) projected
  line L190 (65.6699, -36.4245) -> (70.6699, -45.0848) projected
  line L191 (70.6699, -27.7643) -> (65.6699, -36.4245) projected
  line L192 (80.6699, -27.7643) -> (70.6699, -27.7643) projected
  line L193 (85.6699, -36.4245) -> (80.6699, -27.7643) projected
  line L194 (80.6699, -45.0848) -> (85.6699, -36.4245) projected
  line L195 (70.6699, -45.0848) -> (80.6699, -45.0848) projected
  line L196 (61.3397, -38.9245) -> (51.3397, -38.9245) projected
  line L197 (66.3397, -47.5848) -> (61.3397, -38.9245) projected
  line L198 (61.3397, -56.245) -> (66.3397, -47.5848) projected
  line L199 (51.3397, -56.245) -> (61.3397, -56.245) projected
  line L200 (46.3397, -47.5848) -> (51.3397, -56.245) projected
  line L201 (51.3397, -38.9245) -> (46.3397, -47.5848) projected
  line L202 (27.0096, -36.4245) -> (32.0096, -45.0848) projected
  line L203 (32.0096, -27.7643) -> (27.0096, -36.4245) projected
  line L204 (42.0096, -27.7643) -> (32.0096, -27.7643) projected
  line L205 (47.0096, -36.4245) -> (42.0096, -27.7643) projected
  line L206 (42.0096, -45.0848) -> (47.0096, -36.4245) projected
  line L207 (32.0096, -45.0848) -> (42.0096, -45.0848) projected
  line L208 (-15.981, -38.9245) -> (-25.981, -38.9245) projected
  line L209 (-10.981, -47.5848) -> (-15.981, -38.9245) projected
  line L210 (-15.981, -56.245) -> (-10.981, -47.5848) projected
  line L211 (-25.981, -56.245) -> (-15.981, -56.245) projected
  line L212 (-30.981, -47.5848) -> (-25.981, -56.245) projected
  line L213 (-25.981, -38.9245) -> (-30.981, -47.5848) projected
  line L214 (-11.6509, -36.4245) -> (-6.6509, -45.0848) projected
  line L215 (-6.6509, -27.7643) -> (-11.6509, -36.4245) projected
  line L216 (3.3491, -27.7643) -> (-6.6509, -27.7643) projected
  line L217 (8.3491, -36.4245) -> (3.3491, -27.7643) projected
  line L218 (3.3491, -45.0848) -> (8.3491, -36.4245) projected
  line L219 (-6.6509, -45.0848) -> (3.3491, -45.0848) projected
  line L220 (-50.3111, -36.4245) -> (-45.3111, -45.0848) projected
  line L221 (-45.3111, -27.7643) -> (-50.3111, -36.4245) projected
  line L222 (-35.3111, -27.7643) -> (-45.3111, -27.7643) projected
  line L223 (-30.3111, -36.4245) -> (-35.3111, -27.7643) projected
  line L224 (-35.3111, -45.0848) -> (-30.3111, -36.4245) projected
  line L225 (-45.3111, -45.0848) -> (-35.3111, -45.0848) projected
  line L226 (-54.6413, -38.9245) -> (-64.6413, -38.9245) projected
  line L227 (-49.6413, -47.5848) -> (-54.6413, -38.9245) projected
  line L228 (-54.6413, -56.245) -> (-49.6413, -47.5848) projected
  line L229 (-64.6413, -56.245) -> (-54.6413, -56.245) projected
  line L230 (-69.6413, -47.5848) -> (-64.6413, -56.245) projected
  line L231 (-64.6413, -38.9245) -> (-69.6413, -47.5848) projected
  line L232 (-50.3111, 8.2175) -> (-45.3111, -0.4428) projected
  line L233 (-45.3111, 16.8777) -> (-50.3111, 8.2175) projected
  line L234 (-35.3111, 16.8777) -> (-45.3111, 16.8777) projected
  line L235 (-30.3111, 8.2175) -> (-35.3111, 16.8777) projected
  line L236 (-35.3111, -0.4428) -> (-30.3111, 8.2175) projected
  line L237 (-45.3111, -0.4428) -> (-35.3111, -0.4428) projected
  line L238 (8.3491, 8.2175) -> (3.3491, 16.8777) projected
  line L239 (3.3491, -0.4428) -> (8.3491, 8.2175) projected
  line L240 (-6.6509, -0.4428) -> (3.3491, -0.4428) projected
  line L241 (-11.6509, 8.2175) -> (-6.6509, -0.4428) projected
  line L242 (-6.6509, 16.8777) -> (-11.6509, 8.2175) projected
  line L243 (3.3491, 16.8777) -> (-6.6509, 16.8777) projected
  line L244 (12.6795, 28.038) -> (7.6795, 19.3777) projected
  line L245 (22.6795, 28.038) -> (12.6795, 28.038) projected
  line L246 (27.6795, 19.3777) -> (22.6795, 28.038) projected
  line L247 (22.6795, 10.7175) -> (27.6795, 19.3777) projected
  line L248 (12.6795, 10.7175) -> (22.6795, 10.7175) projected
  line L249 (7.6795, 19.3777) -> (12.6795, 10.7175) projected
  line L250 (42.0096, -0.4428) -> (47.0096, 8.2175) projected
  line L251 (32.0096, -0.4428) -> (42.0096, -0.4428) projected
  line L252 (27.0096, 8.2175) -> (32.0096, -0.4428) projected
  line L253 (32.0096, 16.8777) -> (27.0096, 8.2175) projected
  line L254 (42.0096, 16.8777) -> (32.0096, 16.8777) projected
  line L255 (47.0096, 8.2175) -> (42.0096, 16.8777) projected
  line L256 (70.6699, 16.8777) -> (65.6699, 8.2175) projected
  line L257 (80.6699, 16.8777) -> (70.6699, 16.8777) projected
  line L258 (85.6699, 8.2175) -> (80.6699, 16.8777) projected
  line L259 (80.6699, -0.4428) -> (85.6699, 8.2175) projected
  line L260 (70.6699, -0.4428) -> (80.6699, -0.4428) projected
  line L261 (65.6699, 8.2175) -> (70.6699, -0.4428) projected
  line L262 (105, -25.2638) -> (100, -16.6035) projected
  line L263 (100, -33.924) -> (105, -25.2638) projected
  line L264 (90, -33.924) -> (100, -33.924) projected
  line L265 (85, -25.2638) -> (90, -33.924) projected
  line L266 (90, -16.6035) -> (85, -25.2638) projected
  line L267 (100, -16.6035) -> (90, -16.6035) projected
  line L268 (12.6795, -33.924) -> (22.6795, -33.924) projected
  line L269 (7.6795, -25.2638) -> (12.6795, -33.924) projected
  line L270 (12.6795, -16.6035) -> (7.6795, -25.2638) projected
  line L271 (22.6795, -16.6035) -> (12.6795, -16.6035) projected
  line L272 (27.6795, -25.2638) -> (22.6795, -16.6035) projected
  line L273 (22.6795, -33.924) -> (27.6795, -25.2638) projected
  line L274 (-6.6509, -22.7638) -> (3.3491, -22.7638) projected
  line L275 (-11.6509, -14.1035) -> (-6.6509, -22.7638) projected
  line L276 (-6.6509, -5.4433) -> (-11.6509, -14.1035) projected
  line L277 (3.3491, -5.4433) -> (-6.6509, -5.4433) projected
  line L278 (8.3491, -14.1035) -> (3.3491, -5.4433) projected
  line L279 (3.3491, -22.7638) -> (8.3491, -14.1035) projected
  line L280 (105, -47.5848) -> (100, -38.9245) projected
  line L281 (100, -56.245) -> (105, -47.5848) projected
  line L282 (90, -56.245) -> (100, -56.245) projected
  line L283 (85, -47.5848) -> (90, -56.245) projected
  line L284 (90, -38.9245) -> (85, -47.5848) projected
  line L285 (100, -38.9245) -> (90, -38.9245) projected
  line L286 (12.6795, -56.245) -> (22.6795, -56.245) projected
  line L287 (7.6795, -47.5848) -> (12.6795, -56.245) projected
  line L288 (12.6795, -38.9245) -> (7.6795, -47.5848) projected
  line L289 (22.6795, -38.9245) -> (12.6795, -38.9245) projected
  line L290 (27.6795, -47.5848) -> (22.6795, -38.9245) projected
  line L291 (22.6795, -56.245) -> (27.6795, -47.5848) projected
  line L292 (80.6699, -67.4058) -> (85.6699, -58.7455) projected
  line L293 (70.6699, -67.4058) -> (80.6699, -67.4058) projected
  line L294 (65.6699, -58.7455) -> (70.6699, -67.4058) projected
  line L295 (70.6699, -50.0853) -> (65.6699, -58.7455) projected
  line L296 (80.6699, -50.0853) -> (70.6699, -50.0853) projected
  line L297 (85.6699, -58.7455) -> (80.6699, -50.0853) projected
  line L298 (47.0096, -58.7455) -> (42.0096, -50.0853) projected
  line L299 (42.0096, -67.4058) -> (47.0096, -58.7455) projected
  line L300 (32.0096, -67.4058) -> (42.0096, -67.4058) projected
  line L301 (27.0096, -58.7455) -> (32.0096, -67.4058) projected
  line L302 (32.0096, -50.0853) -> (27.0096, -58.7455) projected
  line L303 (42.0096, -50.0853) -> (32.0096, -50.0853) projected
  line L304 (-6.6509, -67.4058) -> (3.3491, -67.4058) projected
  line L305 (-11.6509, -58.7455) -> (-6.6509, -67.4058) projected
  line L306 (-6.6509, -50.0853) -> (-11.6509, -58.7455) projected
  line L307 (3.3491, -50.0853) -> (-6.6509, -50.0853) projected
  line L308 (8.3491, -58.7455) -> (3.3491, -50.0853) projected
  line L309 (3.3491, -67.4058) -> (8.3491, -58.7455) projected
  line L310 (-35.3111, -67.4058) -> (-30.3111, -58.7455) projected
  line L311 (-45.3111, -67.4058) -> (-35.3111, -67.4058) projected
  line L312 (-50.3111, -58.7455) -> (-45.3111, -67.4058) projected
  line L313 (-45.3111, -50.0853) -> (-50.3111, -58.7455) projected
  line L314 (-35.3111, -50.0853) -> (-45.3111, -50.0853) projected
  line L315 (-30.3111, -58.7455) -> (-35.3111, -50.0853) projected
  line L316 (80.6699, -89.7268) -> (85.6699, -81.0665) projected
  line L317 (70.6699, -89.7268) -> (80.6699, -89.7268) projected
  line L318 (65.6699, -81.0665) -> (70.6699, -89.7268) projected
  line L319 (70.6699, -72.4063) -> (65.6699, -81.0665) projected
  line L320 (80.6699, -72.4063) -> (70.6699, -72.4063) projected
  line L321 (85.6699, -81.0665) -> (80.6699, -72.4063) projected
  line L322 (47.0096, -81.0665) -> (42.0096, -72.4063) projected
  line L323 (42.0096, -89.7268) -> (47.0096, -81.0665) projected
  line L324 (32.0096, -89.7268) -> (42.0096, -89.7268) projected
  line L325 (27.0096, -81.0665) -> (32.0096, -89.7268) projected
  line L326 (32.0096, -72.4063) -> (27.0096, -81.0665) projected
  line L327 (42.0096, -72.4063) -> (32.0096, -72.4063) projected
  line L328 (-6.6509, -89.7268) -> (3.3491, -89.7268) projected
  line L329 (-11.6509, -81.0665) -> (-6.6509, -89.7268) projected
  line L330 (-6.6509, -72.4063) -> (-11.6509, -81.0665) projected
  line L331 (3.3491, -72.4063) -> (-6.6509, -72.4063) projected
  line L332 (8.3491, -81.0665) -> (3.3491, -72.4063) projected
  line L333 (3.3491, -89.7268) -> (8.3491, -81.0665) projected
  line L334 (-35.3111, -89.7268) -> (-30.3111, -81.0665) projected
  line L335 (-45.3111, -89.7268) -> (-35.3111, -89.7268) projected
  line L336 (-50.3111, -81.0665) -> (-45.3111, -89.7268) projected
  line L337 (-45.3111, -72.4063) -> (-50.3111, -81.0665) projected
  line L338 (-35.3111, -72.4063) -> (-45.3111, -72.4063) projected
  line L339 (-30.3111, -81.0665) -> (-35.3111, -72.4063) projected
  line L340 (66.3397, -2.9428) -> (61.3397, 5.7175) projected
  line L341 (61.3397, -11.603) -> (66.3397, -2.9428) projected
  line L342 (51.3397, -11.603) -> (61.3397, -11.603) projected
  line L343 (46.3397, -2.9428) -> (51.3397, -11.603) projected
  line L344 (51.3397, 5.7175) -> (46.3397, -2.9428) projected
  line L345 (61.3397, 5.7175) -> (51.3397, 5.7175) projected
  line L346 (-15.981, 5.7175) -> (-25.981, 5.7175) projected
  line L347 (-10.981, -2.9428) -> (-15.981, 5.7175) projected
  line L348 (-15.981, -11.603) -> (-10.981, -2.9428) projected
  line L349 (-25.981, -11.603) -> (-15.981, -11.603) projected
  line L350 (-30.981, -2.9428) -> (-25.981, -11.603) projected
  line L351 (-25.981, 5.7175) -> (-30.981, -2.9428) projected
  line L352 (-54.6413, 5.7175) -> (-64.6413, 5.7175) projected
  line L353 (-49.6413, -2.9428) -> (-54.6413, 5.7175) projected
  line L354 (-54.6413, -11.603) -> (-49.6413, -2.9428) projected
  line L355 (-64.6413, -11.603) -> (-54.6413, -11.603) projected
  line L356 (-69.6413, -2.9428) -> (-64.6413, -11.603) projected
  line L357 (-64.6413, 5.7175) -> (-69.6413, -2.9428) projected
  line L358 (105, -2.9428) -> (100, 5.7175) projected
  line L359 (100, -11.603) -> (105, -2.9428) projected
  line L360 (90, -11.603) -> (100, -11.603) projected
  line L361 (85, -2.9428) -> (90, -11.603) projected
  line L362 (90, 5.7175) -> (85, -2.9428) projected
  line L363 (100, 5.7175) -> (90, 5.7175) projected
  line L364 (90, 33.038) -> (100, 33.038) projected
  line L365 (85, 41.6983) -> (90, 33.038) projected
  line L366 (90, 50.3585) -> (85, 41.6983) projected
  line L367 (100, 50.3585) -> (90, 50.3585) projected
  line L368 (105, 41.6983) -> (100, 50.3585) projected
  line L369 (100, 33.038) -> (105, 41.6983) projected
  line L370 (-68.9714, 75.1795) -> (-73.9714, 83.8397) projected
  line L371 (-73.9714, 66.5192) -> (-68.9714, 75.1795) projected
  line L372 (-83.9714, 66.5192) -> (-73.9714, 66.5192) projected
  line L373 (-88.9714, 75.1795) -> (-83.9714, 66.5192) projected
  line L374 (-83.9714, 83.8397) -> (-88.9714, 75.1795) projected
  line L375 (-73.9714, 83.8397) -> (-83.9714, 83.8397) projected
  line L376 (-88.3015, -2.9428) -> (-93.3015, 5.7175) projected
  line L377 (-93.3015, -11.603) -> (-88.3015, -2.9428) projected
  line L378 (-103.3015, -11.603) -> (-93.3015, -11.603) projected
  line L379 (-108.3015, -2.9428) -> (-103.3015, -11.603) projected
  line L380 (-103.3015, 5.7175) -> (-108.3015, -2.9428) projected
  line L381 (-93.3015, 5.7175) -> (-103.3015, 5.7175) projected
  line L382 (-108.3015, 19.3777) -> (-103.3015, 10.7175) projected
  line L383 (-103.3015, 28.038) -> (-108.3015, 19.3777) projected
  line L384 (-93.3015, 28.038) -> (-103.3015, 28.038) projected
  line L385 (-88.3015, 19.3777) -> (-93.3015, 28.038) projected
  line L386 (-93.3015, 10.7175) -> (-88.3015, 19.3777) projected
  line L387 (-103.3015, 10.7175) -> (-93.3015, 10.7175) projected
  line L388 (-93.3015, -33.924) -> (-88.3015, -25.2638) projected
  line L389 (-103.3015, -33.924) -> (-93.3015, -33.924) projected
  line L390 (-108.3015, -25.2638) -> (-103.3015, -33.924) projected
  line L391 (-103.3015, -16.6035) -> (-108.3015, -25.2638) projected
  line L392 (-93.3015, -16.6035) -> (-103.3015, -16.6035) projected
  line L393 (-88.3015, -25.2638) -> (-93.3015, -16.6035) projected
  line L394 (-93.3015, -56.245) -> (-88.3015, -47.5848) projected
  line L395 (-103.3015, -56.245) -> (-93.3015, -56.245) projected
  line L396 (-108.3015, -47.5848) -> (-103.3015, -56.245) projected
  line L397 (-103.3015, -38.9245) -> (-108.3015, -47.5848) projected
  line L398 (-93.3015, -38.9245) -> (-103.3015, -38.9245) projected
  line L399 (-88.3015, -47.5848) -> (-93.3015, -38.9245) projected
  line L400 (-103.3015, 77.6795) -> (-93.3015, 77.6795) projected
  line L401 (-108.3015, 86.3397) -> (-103.3015, 77.6795) projected
  line L402 (-103.3015, 95) -> (-108.3015, 86.3397) projected
  line L403 (-93.3015, 95) -> (-103.3015, 95) projected
  line L404 (-88.3015, 86.3397) -> (-93.3015, 95) projected
  line L405 (-93.3015, 77.6795) -> (-88.3015, 86.3397) projected
  line L406 (-108.3014, 41.698) -> (-103.3014, 33.0378) projected
  line L407 (-108.3011, 41.6985) -> (-108.3014, 41.698) projected
  line L408 (-108.3014, 41.6989) -> (-108.3011, 41.6985) projected
  line L409 (-103.3014, 50.3592) -> (-108.3014, 41.6989) projected
  line L410 (-93.3014, 50.3592) -> (-103.3014, 50.3592) projected
  line L411 (-88.3014, 41.6989) -> (-93.3014, 50.3592) projected
  line L412 (-88.3016, 41.6985) -> (-88.3014, 41.6989) projected
  line L413 (-88.3014, 41.698) -> (-88.3016, 41.6985) projected
  line L414 (-93.3014, 33.0378) -> (-88.3014, 41.698) projected
  line L415 (-103.3014, 33.0378) -> (-93.3014, 33.0378) projected
  line L416 (-54.6413, 72.6795) -> (-64.6413, 72.6795) projected
  line L417 (-49.6413, 64.0192) -> (-54.6413, 72.6795) projected